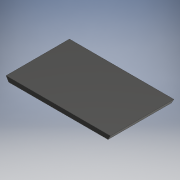
# Autodesk Inventor part: BA14
Saved by Autodesk Inventor 2017 (Build 210142000, 142)
## iProperties
Created: 2019-05-29
Part Number: BA14
Material: Wood (Cherry)
Document SubType Name: Modeling
Designer: Dell
Density: 0.63 g/cm^3
Appearance: Smooth - Black
Author: Dell
Autodesk Inventor part; units mm, degrees
ref_plane "YZ Plane" through (0, 0, 0) normal (1, 0, 0) x (0, 1, 0)
ref_plane "XZ Plane" through (0, 0, 0) normal (0, 1, 0) x (-1, 0, 0)
ref_plane "XY Plane" through (0, 0, 0) normal (0, 0, 1) x (1, 0, 0)
sketch "Sketch1" plane through (0, 0, 0) normal (0, 0, 1) x (1, 0, 0)
  line L0 (0, 0) -> (303.5647, 0)
  line L1 (303.5647, 0) -> (303.5647, 184.15)
  line L2 (303.5647, 184.15) -> (0, 184.15)
  line L3 (0, 184.15) -> (0, 0)
  dimension "d0" = 303.5647
  dimension "d1" = 184.15
  constraints: 8 end point, 2 parallel, 1 horizontal, 1 perpendicular
  measures "d0" distance of L0.start L0.end
  measures "d1" distance of L2.end L0.start
extrude "Extrusion1" add sketch "Sketch1" along normal blind 12.7
sketch "Sketch2" plane through (0, 184.15, 0) normal (0, 1, 0) x (1, 0, 0)
  line L0 (0, -12.7) -> (303.5647, -12.7) projected
  line L1 (0, -12.7) -> (7.3323, 0)
  line L2 (7.3323, 0) -> (0, 0)
  line L3 (0, 0) -> (0, -12.7)
  line L4 (0, 0) -> (303.5647, 0) projected
  line L5 (303.5647, 0) -> (303.5647, -12.7) projected
  line L6 (296.2324, 0) -> (303.5647, -12.7)
  line L7 (303.5647, -12.7) -> (303.5647, 0)
  line L8 (303.5647, 0) -> (296.2324, 0)
  dimension "d4" = 30
  dimension "d5" = 30
  constraints: 12 end point, 2 perpendicular, 1 collinear, 1 parallel, 1 point on line
  measures "d4" angle of L5 L6
  measures "d5" angle of L3 L1
extrude "Extrusion2" cut sketch "Sketch2" against normal through all contours L3 L2 L1 | L6 L4 L5
body "Solid1"
